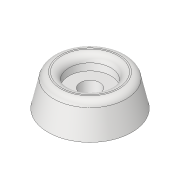
# Autodesk Inventor part: FOOT
Saved by Autodesk Inventor 2020 (Build 240168000, 168)
## iProperties
Created: 2020-04-13
Part Number: FOOT
Material: Generic
Document SubType Name: Modeling
Designer: John K
Density: 1 g/cm^3
Appearance: Default
Description: McM 9540K59
Author: John K
Autodesk Inventor part; units mm, degrees
ref_plane "YZ Plane" through (0, 0, 0) normal (1, 0, 0) x (0, 1, 0)
ref_plane "XZ Plane" through (0, 0, 0) normal (0, 1, 0) x (-1, 0, 0)
ref_plane "XY Plane" through (0, 0, 0) normal (0, 0, 1) x (1, 0, 0)
sketch "Sketch1" plane through (0, 0, 0) normal (0, 0, 1) x (1, 0, 0)
  line L0 (-2.3813, 3.9688) -> (-4.7625, 3.9688)
  line L1 (-4.7625, 3.9688) -> (-4.7625, 8.7313)
  line L2 (-4.7625, 8.7313) -> (-9.525, 8.7312)
  line L3 (-9.525, 8.7312) -> (-12.3031, 0)
  line L4 (-12.3031, 0) -> (-2.3812, 0)
  line L5 (0, 0) -> (0, -4.1368)
  line L6 (-2.3813, 3.9688) -> (-2.3812, 0)
  dimension "d0" = 9.525
  dimension "d1" = 24.6062
  dimension "d2" = 3.9688
  dimension "d3" = 4.7625
  dimension "d4" = 8.7312
  dimension "d5" = 4.7625
  constraints: 14 end point, 3 perpendicular, 1 horizontal, 1 horizontal alignment, 1 parallel, 1 vertical
  measures "d0" diameter of L1 L5
  measures "d1" diameter of L3.end L5
  measures "d2" distance between parallel lines of L4 L0
  measures "d3" diameter of L6 L5
  measures "d4" distance between parallel lines of L2 L4
  measures "d5" distance of L1.end L2.end
revolve "Revolution1" add sketch "Sketch1" angle 360 about axis through (0, 0, 0) along (0, -1, 0)
fillet "Fillet1" radius 1.5875 2 edges at (9.525, 8.7312, 0) (4.7625, 8.7313, 0)
body "Solid1"
